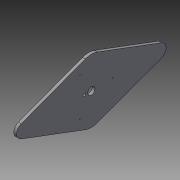
# Autodesk Inventor part: RibSimple
Saved by Autodesk Inventor 2014 SP1 (Build 180222100, 222)
## iProperties
Created: 2014-11-10
Part Number: RibSimple
Material: Generic
Document SubType Name: Modeling
Designer: rawrdong
Density: 1 g/cm^3
Appearance: Default
Author: rawrdong
Autodesk Inventor part; units mm, degrees
ref_plane "YZ Plane" through (0, 0, 0) normal (1, 0, 0) x (0, 1, 0)
ref_plane "XZ Plane" through (0, 0, 0) normal (0, 1, 0) x (-1, 0, 0)
ref_plane "XY Plane" through (0, 0, 0) normal (0, 0, 1) x (1, 0, 0)
sketch "Sketch1" plane through (0, 0, 0) normal (1, 0, 0) x (0, 1, 0)
  line L0 (-122.5, 0) -> (122.5, 0) construction
  line L1 (0, -52.5) -> (0, 52.5) construction
  line L2 (-100, 0) -> (0, 37.5)
  line L3 (0, 37.5) -> (100, 0)
  line L4 (100, 0) -> (0, -37.5)
  line L5 (-100, 0) -> (0, -37.5)
  circle A0 centre (0, 0) radius 4.175
  circle A1 centre (25, 0) radius 0.75
  line L6 (25, 0) -> (-12.5, -21.6506) construction
  line L7 (-12.5, -21.6506) -> (-12.5, 21.6506) construction
  line L8 (-12.5, 21.6506) -> (25, 0) construction
  circle A2 centre (-12.5, 21.6506) radius 0.75
  circle A3 centre (-12.5, -21.6506) radius 0.75
  circle A4 centre (0, 0) radius 25 construction
  dimension "d7" = 50
  dimension "d3" = 8.35
  dimension "d4" = 1.5
  dimension "d11" = 75
  dimension "d24" = 200
  constraints: 14 end point, 5 coincident, 5 point on line, 4 centre point, 2 equal radius, 1 parallel, 11 other
  measures "d3" diameter of A0
  measures "d4" diameter of A1
  measures "d11" distance of L2.end L4.end
  measures "d24" distance of L3.end L2.start
extrude "Extrusion1" add sketch "Sketch1" along normal blind 3.2
fillet "Fillet1" radius 20 2 edges at (1.6, 0, 37.5) (1.6, 0, -37.5)
sketch "Sketch4" plane through (3.2, 0, 0) normal (1, 0, 0) x (0, 0, -1)
  circle A0 centre (0, 0) radius 4.175 projected
  circle A1 centre (0, -7.9) radius 1.425
  dimension "d20" = 7.9
  dimension "d21" = 2.85
  constraints: 1 centre point, 1 vertical alignment
  measures "d20" distance of A1.centre A0.centre
  measures "d21" diameter of A1
extrude "Extrusion4" cut sketch "Sketch4" against normal through all contours A1
fillet "Fillet4" radius 8 2 edges at (1.6, 100, 0) (1.6, -100, 0)
sketch "Sketch5" plane through (0, 0, 0) normal (-1, 0, 0) x (0, 0, 1)
  circle A0 centre (-21.6506, -12.5) radius 0.75 projected
  circle A1 centre (-2.0715, -16.5813) radius 1.425
  line L0 (-2.0715, -16.5813) -> (-21.6506, -12.5) construction
  circle A2 centre (0, -7.9) radius 1.425 projected
  circle A3 centre (0, 0) radius 4.175 projected
  circle A4 centre (-2.0715, -16.5813) radius 7.5 construction
  line L1 (-2.0715, -16.5813) -> (7.7181, -18.6219) construction
  circle A5 centre (7.7181, -18.6219) radius 1.425
  circle A6 centre (15.3955, 6.4967) radius 1.425
  circle A7 centre (12.268, 15.995) radius 1.425
  circle A8 centre (-13.3241, 10.0846) radius 1.425
  circle A9 centre (-19.9861, 2.6269) radius 1.425
  point P0 (22.1831, -13.0282)
  point P1 (-22.1831, -13.0282)
  dimension "d31" = 2.85
  dimension "d32" = 20
  dimension "d33" = 15
  dimension "d38" = 10
  dimension "d41" = 360
  constraints: 7 centre point, 4 end point, 2 coincident, 1 collinear, 1 equal radius, 1 tangent, 14 other
  measures "d31" diameter of A1
  measures "d32" distance of L0.start L0.end
  measures "d33" diameter of A4
  measures "d38" distance of L1.start L1.end
sketch "Sketch3" plane through (3.2, 0, 0) normal (1, 0, 0) x (0, 0, -1)
  line L0 (-7.7286, 24.361) -> (0, 66.8014)
  line L1 (0, 66.8014) -> (7.7286, 24.361)
  line L2 (8.0286, -24.361) -> (0, -68.4486)
  line L3 (0, -68.4486) -> (-8.0286, -24.361)
  line L4 (-7.7286, 24.361) -> (7.7286, 24.361)
  line L5 (-8.0286, -24.361) -> (8.0286, -24.361)
  line L6 (52.5, 0) -> (-52.5, 0) projected
  constraints: 12 end point, 1 horizontal, 1 parallel, 1 other
sketch "Sketch2" plane through (3.2, 0, 0) normal (1, 0, 0) x (0, 0, -1)
  circle A0 centre (0, 0) radius 4.175 projected
  circle A1 centre (0, 0) radius 3.048
  dimension "d13" = 6.096
  constraints: 1 centre point, 1 coincident
  measures "d13" diameter of A1
equation "\"d24\" = Height"
equation "\"Height\" = 200"
body "Solid1"
